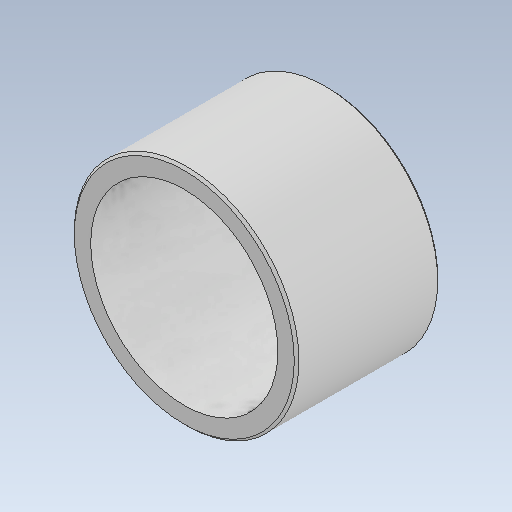
# Autodesk Inventor part: Peça44
Saved by Autodesk Inventor 2021 (Build 250183000, 183)
## iProperties
Category: 41
Created: 2021-07-25
Part Number: Peça44
Material: Genérico
Document SubType Name: Modeling
Designer: Giovanni
Density: 1 g/cm^3
Appearance: Padrão
User Status: 1:1
Author: Giovanni
Keywords: 40
Autodesk Inventor part; units mm, degrees
ref_plane "YZ Plane" through (0, 0, 0) normal (1, 0, 0) x (0, 1, 0)
ref_plane "XZ Plane" through (0, 0, 0) normal (0, 1, 0) x (-1, 0, 0)
ref_plane "XY Plane" through (0, 0, 0) normal (0, 0, 1) x (1, 0, 0)
sketch "Esboço1" plane through (0, 0, 0) normal (0, 0, 1) x (1, 0, 0)
  circle A0 centre (0, 0) radius 20
  circle A1 centre (0, 0) radius 24
  dimension "d0" = 40
  dimension "d1" = 48
  constraints: 2 centre point, 2 coincident
  measures "d0" diameter of A0
  measures "d1" diameter of A1
extrude "Extrusão1" add sketch "Esboço1" along normal mid plane 30.65
chamfer "Chanfro1" distance 0.5 angle 45 2 edges at (-24, 0, 15.325) (-24, 0, -15.325)
